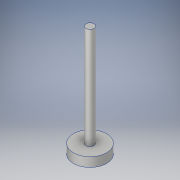
# Autodesk Inventor part: Embolo
Saved by Autodesk Inventor 2019 (Build 230136000, 136)
## iProperties
Created: 2019-09-21
Part Number: Embolo
Material: Aluminio 6061
Document SubType Name: Modeling
Designer: axelj
Density: 2.7 g/cm^3
Appearance: Aluminio - Plano
Author: axelj
Autodesk Inventor part; units mm, degrees
ref_plane "YZ Plane" through (0, 0, 0) normal (1, 0, 0) x (0, 1, 0)
ref_plane "XZ Plane" through (0, 0, 0) normal (0, 1, 0) x (-1, 0, 0)
ref_plane "XY Plane" through (0, 0, 0) normal (0, 0, 1) x (1, 0, 0)
sketch "Boceto1" plane through (0, 0, 0) normal (0, 1, 0) x (-1, 0, 0)
  circle A0 centre (0, 0) radius 1.45
  dimension "d0" = 2.9
  constraints: 1 centre point, 1 coincident
  measures "d0" diameter of A0
extrude "Extrusión1" add sketch "Boceto1" against normal blind 30.7
sketch "Boceto2" plane through (0, -30.7, 0) normal (0, -1, 0) x (1, 0, 0)
  circle A0 centre (0, 0) radius 5.9
  dimension "d3" = 11.8
  constraints: 1 centre point, 1 coincident
  measures "d3" diameter of A0
extrude "Extrusión2" add sketch "Boceto2" along normal blind 3.3
sketch "Boceto3" plane through (0, 0, 0) normal (0, 1, 0) x (1, 0, 0)
  circle A0 centre (0, 0) radius 1.45 projected
  circle A1 centre (0, 0) radius 1.45
  dimension "d6" = 2.9
  constraints: 1 centre point, 1 coincident
  measures "d6" diameter of A1
extrude "Extrusión3" add sketch "Boceto3" along normal blind 5.4
